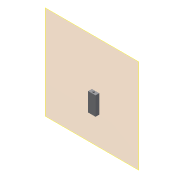
# Autodesk Inventor part: Motor
Saved by Autodesk Inventor 2017 (Build 210142000, 142)
## iProperties
Created: 2017-03-11
Part Number: Motor
Material: Generic
Document SubType Name: Modeling
Designer: zallen
Density: 1 g/cm^3
Appearance: Default
Author: zallen
Autodesk Inventor part; units mm, degrees
ref_plane "YZ Plane" through (0, 0, 0) normal (1, 0, 0) x (0, 1, 0)
ref_plane "XZ Plane" through (0, 0, 0) normal (0, 1, 0) x (-1, 0, 0)
ref_plane "XY Plane" through (0, 0, 0) normal (0, 0, 1) x (1, 0, 0)
ref_plane "Work Plane1" through (403.2389, 230.5529, 0) normal (0, 0, 1) x (0.3695663, 0.9292043, 0)
sketch "Sketch1" plane through (403.2389, 230.5529, 0) normal (0, 0, 1) x (0.3695663, 0.9292043, 0)
  line L0 (-363.2543, 289.4868) -> (-312.4543, 289.4868)
  line L1 (-312.4543, 289.4868) -> (-312.4543, 162.4868)
  line L2 (-312.4543, 162.4868) -> (-363.2543, 162.4868)
  line L3 (-363.2543, 162.4868) -> (-363.2543, 289.4868)
  dimension "d0" = 50.8
  dimension "d1" = 127
  constraints: 8 end point, 2 parallel, 1 horizontal, 1 perpendicular
  measures "d0" distance of L1.end L2.end
  measures "d1" distance of L0.end L1.end
extrude "Extrusion1" add sketch "Sketch1" along normal blind 25.4
sketch "Sketch2" plane through (0, 0, 0) normal (-0.9292043, 0.3695663, 0) x (0.3695663, 0.9292043, 0)
  circle A0 centre (25.4, -12.7) radius 6.35
  line L0 (0, 0) -> (0, -25.4) projected
  line L1 (50.8, -25.4) -> (0, -25.4) projected
  dimension "d4" = 12.7
  dimension "d5" = 25.4
  dimension "d6" = 12.7
  constraints: 1 centre point
  measures "d4" diameter of A0
  measures "d5" distance from line of L0 A0.centre
  measures "d6" distance from line of L1 A0.centre
extrude "Extrusion2" add sketch "Sketch2" along normal blind 6.35
body "Solid1"
